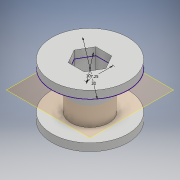
# Autodesk Inventor part: movingSpindle
Saved by Autodesk Inventor 2018 (Build 220112000, 112)
## iProperties
Created: 2018-11-25
Part Number: movingSpindle
Material: Generic
Document SubType Name: Modeling
Designer: Prakash
Density: 1 g/cm^3
Appearance: Default
Author: Prakash
Autodesk Inventor part; units mm, degrees
ref_plane "YZ Plane" through (0, 0, 0) normal (1, 0, 0) x (0, 1, 0)
ref_plane "XZ Plane" through (0, 0, 0) normal (0, 1, 0) x (-1, 0, 0)
ref_plane "XY Plane" through (0, 0, 0) normal (0, 0, 1) x (1, 0, 0)
sketch "Sketch1" plane through (0, 0, 0) normal (0, 0, 1) x (1, 0, 0)
  circle A0 centre (0, 0) radius 10
  circle A1 centre (0, 0) radius 5
  line L0 (4.1858, 0) -> (2.0929, -3.625)
  line L1 (2.0929, -3.625) -> (-2.0929, -3.625)
  line L2 (-2.0929, -3.625) -> (-4.1858, 0)
  line L3 (-4.1858, 0) -> (-2.0929, 3.625)
  line L4 (-2.0929, 3.625) -> (2.0929, 3.625)
  line L5 (2.0929, 3.625) -> (4.1858, 0)
  dimension "d1" = 20
  dimension "d2" = 10
  dimension "d3" = 7.25
  constraints: 12 end point, 3 coincident, 2 centre point, 1 horizontal, 13 other
  measures "d1" diameter of A0
  measures "d2" diameter of A1
  measures "d3" distance between parallel lines of L1 L4
extrude "Extrusion2" add sketch "Sketch1" against normal blind 10 contours A1
sketch "Sketch3" plane through (0, 0, -10) normal (0, 0, -1) x (-1, 0, 0)
  circle A0 centre (0, 0) radius 10 projected
  circle A1 centre (0, 0) radius 5 projected
  line L0 (-2.0929, 3.625) -> (-4.1858, 0) projected
  line L1 (-4.1858, 0) -> (-2.0929, -3.625) projected
  line L2 (-2.0929, -3.625) -> (2.0929, -3.625) projected
  line L3 (2.0929, -3.625) -> (4.1858, 0) projected
  line L4 (4.1858, 0) -> (2.0929, 3.625) projected
  line L5 (2.0929, 3.625) -> (-2.0929, 3.625) projected
extrude "Extrusion3" add sketch "Sketch3" along normal blind 2 contours A0 | A1
extrude "Extrusion4" add sketch "Sketch1" along normal blind 2 contours A0 | A1
ref_plane "Work Plane1" through (0, 0, -5) normal (0, 0, 1) x (1, 0, 0)
sketch "Sketch4" plane through (0, 0, -5) normal (0, 0, 1) x (1, 0, 0)
  circle A0 centre (0, 0) radius 5 projected
  arc A1 (1.5, 4.7697) -> (-1.5, 4.7697) centre (0, 0) ccw
  line L0 (0, 0) -> (0, 5) construction
  line L1 (-1.5, 4.7697) -> (-1.5, 9.7697)
  line L2 (-1.5, 9.7697) -> (1.5, 9.7697)
  line L3 (1.5, 9.7697) -> (1.5, 4.7697)
  dimension "d12" = 5
  dimension "d13" = 3
  constraints: 8 end point, 6 point on circle, 3 vertical, 1 centre point, 1 perpendicular
  measures "d12" distance of L1.start L1.end
  measures "d13" distance of L1.end L2.end
extrude "Extrusion5" add sketch "Sketch4" along normal mid plane 3 contours A0 L1 L2 L3
body "Solid1"
